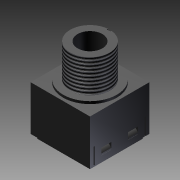
# Autodesk Inventor part: tl-cap
Saved by Autodesk Inventor 2011 SP1 (Build 150282100, 282)
## iProperties
Created: 2013-12-24
Part Number: tl-cap
Catalog Web Link: www.cadenas.de
Description: TL Series - Fully Illuminated Toggles - body-
Vendor: NKKSWITCHES
Document SubType Name: Modeling
Designer: PARTuser1
Manufacturer: NKKSWITCHES
Density: 1 g/cm^3
Category: PARTsolutions
Company: NKKSWITCHES
Title: tl-cap
Author: Cadenas PARTsolutions
PSOL_IDENT_0: {$CADENAS_DATA\23d-libs\nkkswitches\toggle\tl\parts\tl_body.prj},192 {VTYP=3D},{NB=tl-cap},{LINA=tl-
PSOL_IDENT_1: cap},{NN=TL Series - Fully Illuminated Toggles - body},{DATE=08.04.2009 12:11:38},{GEOMDATE=26.03.20
PSOL_IDENT_2: 09 10:58:00},{VERSION=},{LINEID=10},{LINESUBID=-1},{WBVAR=}  {NB=tl-cap},{LINA=tl-cap},{KT=DUMMY},{S
PSOL_IDENT_3: RS=TL},{PN=tl-cap},{ND=12},{PITCH=1}
CNS_NN: TL Series - Fully Illuminated Toggles - body
CNS_NB: tl-cap
CNS_NBSYN: $PN.
CNS_LINA: tl-cap
CNS_SRS: TL
CNS_PN: tl-cap
CNS_ND: 12.000
CNS_PITCH: 1.000
SUPPLIER: NKKSWITCHES
ARTICLENO: tl-cap
BOMINFO: tl-cap
CREATOR: CADENAS GmbH
Autodesk Inventor part; units mm, degrees
sketch "Sketch_1" plane through (0, 0, 0) normal (1, 0, 0) x (0, 1, 0)
  line L0 (0, 9.0043) -> (-15.5956, 9.0043)
  line L1 (-15.5956, 9.0043) -> (-15.5956, -9.0043)
  line L2 (-15.5956, -9.0043) -> (0, -9.0043)
  line L3 (0, -9.0043) -> (0, 9.0043)
  constraints: 8 end point
extrude "Extrusion1" add sketch "Sketch_1" along normal mid plane 18.0086
sketch "Sketch_2" plane through (0, 0, 0) normal (0, 1, 0) x (-1, 0, 0)
  line L0 (12.2936, -12.2936) -> (12.2936, 12.2936)
  line L1 (12.2936, 12.2936) -> (-12.2936, 12.2936)
  line L2 (-12.2936, 12.2936) -> (-12.2936, -12.2936)
  line L3 (-12.2936, -12.2936) -> (12.2936, -12.2936)
  circle A0 centre (0, 0) radius 8.128
  constraints: 8 end point, 1 centre point
extrude "Extrusion2" cut sketch "Sketch_2" along normal mid plane 1.524
sketch "Sketch_3" plane through (0, -15.5956, 0) normal (0, 1, 0) x (1, 0, 0)
  line L0 (-11.5316, 11.5316) -> (-11.5316, -11.5316)
  line L1 (-11.5316, -11.5316) -> (11.5316, -11.5316)
  line L2 (11.5316, -11.5316) -> (11.5316, 11.5316)
  line L3 (11.5316, 11.5316) -> (-11.5316, 11.5316)
  line L4 (-7.9883, 7.9883) -> (-7.9883, -7.9883)
  line L5 (-7.9883, -7.9883) -> (7.9883, -7.9883)
  line L6 (7.9883, -7.9883) -> (7.9883, 7.9883)
  line L7 (7.9883, 7.9883) -> (-7.9883, 7.9883)
  constraints: 16 end point
extrude "Extrusion3" cut sketch "Sketch_3" along normal mid plane 2.54
sketch "Sketch_4" plane through (0, -14.3256, 0) normal (0, 1, 0) x (1, 0, 0)
  line L0 (-12.446, 12.446) -> (-12.446, -12.446)
  line L1 (-12.446, -12.446) -> (12.446, -12.446)
  line L2 (12.446, -12.446) -> (12.446, 12.446)
  line L3 (12.446, 12.446) -> (-12.446, 12.446)
  line L4 (-11.5316, -7.5692) -> (-7.9883, -7.5692)
  line L5 (-7.9883, -7.5692) -> (-7.9883, -7.874)
  line L6 (-7.9883, -7.874) -> (-11.5316, -7.874)
  line L7 (-11.5316, -7.874) -> (-11.5316, -11.5316)
  line L8 (-11.5316, -11.5316) -> (11.5316, -11.5316)
  line L9 (11.5316, -11.5316) -> (11.5316, -7.874)
  line L10 (11.5316, -7.874) -> (7.9883, -7.874)
  line L11 (7.9883, -7.874) -> (7.9883, -7.5692)
  line L12 (7.9883, -7.5692) -> (11.5316, -7.5692)
  line L13 (11.5316, -7.5692) -> (11.5316, 7.5692)
  line L14 (11.5316, 7.5692) -> (7.9883, 7.5692)
  line L15 (7.9883, 7.5692) -> (7.9883, 7.874)
  line L16 (7.9883, 7.874) -> (11.5316, 7.874)
  line L17 (11.5316, 7.874) -> (11.5316, 11.5316)
  line L18 (11.5316, 11.5316) -> (-11.5316, 11.5316)
  line L19 (-11.5316, 11.5316) -> (-11.5316, 7.874)
  line L20 (-11.5316, 7.874) -> (-7.9883, 7.874)
  line L21 (-7.9883, 7.874) -> (-7.9883, 7.5692)
  line L22 (-7.9883, 7.5692) -> (-11.5316, 7.5692)
  line L23 (-11.5316, 7.5692) -> (-11.5316, -7.5692)
  constraints: 48 end point
extrude "Extrusion4" cut sketch "Sketch_4" along normal mid plane 10.16
sketch "Sketch_5" plane through (0, -14.3256, 0) normal (0, 1, 0) x (1, 0, 0)
  line L0 (-7.7343, 7.7343) -> (-7.7343, -7.7343)
  line L1 (-7.7343, -7.7343) -> (7.7343, -7.7343)
  line L2 (7.7343, -7.7343) -> (7.7343, 7.7343)
  line L3 (7.7343, 7.7343) -> (-7.7343, 7.7343)
  constraints: 8 end point
extrude "Extrusion5" add sketch "Sketch_5" against normal blind 1.2954
sketch "Sketch_6" plane through (9.0043, 0, 0) normal (1, 0, 0) x (0, 0, -1)
  line L0 (2.54, -10.668) -> (2.54, -12.7)
  line L1 (2.54, -12.7) -> (5.588, -12.7)
  line L2 (5.588, -12.7) -> (5.588, -10.668)
  line L3 (5.588, -10.668) -> (2.54, -10.668)
  constraints: 8 end point
extrude "Extrusion6" cut sketch "Sketch_6" against normal blind 18.0086
sketch "Sketch_7" plane through (9.0043, 0, 0) normal (1, 0, 0) x (0, 0, -1)
  line L0 (-5.588, -10.668) -> (-5.588, -12.7)
  line L1 (-5.588, -12.7) -> (-2.54, -12.7)
  line L2 (-2.54, -12.7) -> (-2.54, -10.668)
  line L3 (-2.54, -10.668) -> (-5.588, -10.668)
  constraints: 8 end point
extrude "Extrusion7" cut sketch "Sketch_7" against normal blind 18.0086
sketch "Sketch_8" plane through (0, 0, 4.064) normal (0, 0, 1) x (1, 0, 0)
  line L0 (-9.0043, -12.6492) -> (-8.9535, -12.6492)
  line L1 (-8.9535, -12.6492) -> (-8.9535, -12.7)
  line L2 (-8.9535, -12.7) -> (8.9535, -12.7)
  line L3 (8.9535, -12.7) -> (8.9535, -12.6492)
  line L4 (8.9535, -12.6492) -> (9.0043, -12.6492)
  line L5 (9.0043, -12.6492) -> (9.0043, -12.192)
  arc A0 (9.0043, -12.192) -> (7.7343, -11.176) centre (6.8661, -13.563) ccw
  line L6 (7.7343, -11.176) -> (7.7343, -10.668)
  line L7 (7.7343, -10.668) -> (-7.7343, -10.668)
  line L8 (-7.7343, -10.668) -> (-7.7343, -11.176)
  arc A1 (-7.7343, -11.176) -> (-9.0043, -12.192) centre (-6.8661, -13.563) ccw
  line L9 (-9.0043, -12.192) -> (-9.0043, -12.6492)
  constraints: 20 end point, 4 point on circle, 2 centre point
extrude "Extrusion8" add sketch "Sketch_8" along normal mid plane 2.9972
sketch "Sketch_9" plane through (0, 0, -4.064) normal (0, 0, 1) x (1, 0, 0)
  line L0 (-9.0043, -12.6492) -> (-8.9535, -12.6492)
  line L1 (-8.9535, -12.6492) -> (-8.9535, -12.7)
  line L2 (-8.9535, -12.7) -> (8.9535, -12.7)
  line L3 (8.9535, -12.7) -> (8.9535, -12.6492)
  line L4 (8.9535, -12.6492) -> (9.0043, -12.6492)
  line L5 (9.0043, -12.6492) -> (9.0043, -12.192)
  arc A0 (9.0043, -12.192) -> (7.7343, -11.176) centre (6.8661, -13.563) ccw
  line L6 (7.7343, -11.176) -> (7.7343, -10.668)
  line L7 (7.7343, -10.668) -> (-7.7343, -10.668)
  line L8 (-7.7343, -10.668) -> (-7.7343, -11.176)
  arc A1 (-7.7343, -11.176) -> (-9.0043, -12.192) centre (-6.8661, -13.563) ccw
  line L9 (-9.0043, -12.192) -> (-9.0043, -12.6492)
  constraints: 20 end point, 4 point on circle, 2 centre point
extrude "Extrusion9" add sketch "Sketch_9" along normal mid plane 2.9972
sketch "Sketch_11" plane through (0, 0, 0) normal (1, 0, 0) x (0, 1, 0)
  line L0 (0, 0) -> (10.0076, 0)
  line L1 (0, -3.7592) -> (0, -6)
  line L2 (0, -6) -> (10.0076, -6)
  line L3 (10.0076, -6) -> (10.0076, -3.7592)
  line L4 (10.0076, -3.7592) -> (0, -3.7592)
  constraints: 10 end point
revolve "Revolution1" add sketch "Sketch_11" angle 360 about axis through (0, 0, 0) along (0, -1, 0)
thread "Thread1" size "M12x1" class "6g" standard "ISO Metric profile" full length
sketch "Sketch_15" plane through (0, 0, 0) normal (0, 1, 0) x (-1, 0, 0)
  line L0 (0.508, -5.6444) -> (-0.508, -5.6444)
  line L1 (-0.508, -5.6444) -> (-0.508, -6.4064)
  line L2 (-0.508, -6.4064) -> (0.508, -6.4064)
  line L3 (0.508, -6.4064) -> (0.508, -5.6444)
  constraints: 8 end point
extrude "Extrusion10" cut sketch "Sketch_15" along normal blind 50.8
sketch "Sketch_18" plane through (0, 0, 0) normal (1, 0, 0) x (0, 1, 0)
  line L0 (0, 0) -> (1.27, 0)
  line L1 (1.27, 0) -> (1.27, -6)
  line L2 (1.27, -6) -> (0, -6)
  line L3 (0, -6) -> (0, 0)
  line L4 (0, 0) -> (1.27, 0)
  constraints: 10 end point
revolve "Revolution2" add sketch "Sketch_18" angle 360 about axis through (0, 0, 0) along (0, -1, 0)
ref_plane "body_to_dummy_XY" through (0, 0, 0) normal (0, 1, 0) x (1, 0, 0)
ref_plane "body_to_dummy_YZ" through (0, 0, 0) normal (1, 0, 0) x (0, 0, -1)
ref_plane "body_to_dummy_ZX" through (0, 0, 0) normal (0, 0, -1) x (0, 1, 0)
ref_plane "body_to_hex_nut_XY" through (0, 0, 0) normal (0, 1, 0) x (1, 0, 0)
ref_plane "body_to_hex_nut_YZ" through (0, 0, 0) normal (1, 0, 0) x (0, 0, -1)
ref_plane "body_to_hex_nut_ZX" through (0, 0, 0) normal (0, 0, -1) x (0, 1, 0)
ref_plane "body_to_hex_nut_black_XY" through (0, 2.5146, 0) normal (0, 1, 0) x (1, 0, 0)
ref_plane "body_to_hex_nut_black_YZ" through (0, 2.5146, 0) normal (1, 0, 0) x (0, 0, -1)
ref_plane "body_to_hex_nut_black_ZX" through (0, 2.5146, 0) normal (0, 0, -1) x (0, 1, 0)
ref_plane "body_to_lockwasher_XY" through (0, 2.0066, 0) normal (0, 1, 0) x (1, 0, 0)
ref_plane "body_to_lockwasher_YZ" through (0, 2.0066, 0) normal (1, 0, 0) x (0, 0, -1)
ref_plane "body_to_lockwasher_ZX" through (0, 2.0066, 0) normal (0, 0, -1) x (0, 1, 0)
ref_plane "body_to_pins_XY" through (0, -15.5956, 0) normal (0, 1, 0) x (1, 0, 0)
ref_plane "body_to_pins_YZ" through (0, -15.5956, 0) normal (1, 0, 0) x (0, 0, -1)
ref_plane "body_to_pins_ZX" through (0, -15.5956, 0) normal (0, 0, -1) x (0, 1, 0)
ref_plane "body_to_toggles_XY" through (0, 10.0076, 0) normal (0, -1, 0) x (1, 0, 0)
ref_plane "body_to_toggles_YZ" through (0, 10.0076, 0) normal (1, 0, 0) x (0, 0, 1)
ref_plane "body_to_toggles_ZX" through (0, 10.0076, 0) normal (0, 0, 1) x (0, -1, 0)
body "Solid1"
